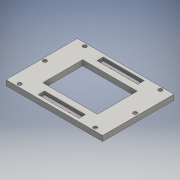
# Autodesk Inventor part: modified_xyStageMount
Saved by Autodesk Inventor 2016 (Build 200138000, 138)
## iProperties
Created: 2016-09-14
Part Number: modified_xyStageMount
Material: Generic
Document SubType Name: Modeling
Designer: sims01
Density: 1 g/cm^3
Appearance: Default
Author: sims01
Autodesk Inventor part; units mm, degrees
ref_plane "YZ Plane" through (0, 0, 0) normal (1, 0, 0) x (0, 1, 0)
ref_plane "XZ Plane" through (0, 0, 0) normal (0, 1, 0) x (-1, 0, 0)
ref_plane "XY Plane" through (0, 0, 0) normal (0, 0, 1) x (1, 0, 0)
sketch "Sketch1" plane through (0, 0, 0) normal (0, 0, 1) x (1, 0, 0)
  line L0 (-230, 170) -> (230, 170)
  line L1 (230, 170) -> (230, -170)
  line L2 (230, -170) -> (-230, -170)
  line L3 (-230, -170) -> (-230, 170)
  line L4 (130, 170) -> (230, 170)
  line L5 (230, 170) -> (230, -170)
  line L6 (230, -170) -> (130, -170)
  line L7 (130, -170) -> (130, 170)
  line L8 (-230, 170) -> (-130, 170)
  line L9 (-130, 170) -> (-130, -170)
  line L10 (-130, -170) -> (-230, -170)
  line L11 (-230, -170) -> (-230, 170)
  line L12 (-230, 170) -> (230, 170)
  line L13 (230, 170) -> (230, 95)
  line L14 (230, 95) -> (-230, 95)
  line L15 (-230, 95) -> (-230, 170)
  line L16 (-230, -95) -> (230, -95)
  line L17 (230, -95) -> (230, -170)
  line L18 (230, -170) -> (-230, -170)
  line L19 (-230, -170) -> (-230, -95)
  point P0 (0, 0)
  dimension "d0" = 460
  dimension "d1" = 340
  dimension "d2" = 170
  dimension "d3" = 230
  dimension "d4" = 100
  dimension "d5" = 100
  dimension "d6" = 75
  dimension "d7" = 75
  constraints: 40 end point, 12 collinear, 10 parallel, 5 horizontal, 5 perpendicular
  measures "d0" distance of L0.start L0.end
  measures "d1" distance of L0.end L1.end
  measures "d2" distance from line of point (0, 0) L0
  measures "d3" distance from line of point (0, 0) L1
  measures "d4" distance of L4.start L4.end
  measures "d5" distance of L8.start L8.end
  measures "d6" distance between parallel lines of L2 L16
  measures "d7" distance between parallel lines of L14 L0
extrude "Extrusion1" add sketch "Sketch1" along normal blind 25 contours L0 L9 L14 L3 | L0 L7 L14 L9 | L14 L9 L16 L3 | L0 L1 L14 L7 | L16 L9 L2 L3 | L14 L1 L16 L7 | L16 L7 L2 L9 | L16 L1 L2 L7
sketch "Sketch2" plane through (0, 0, 25) normal (0, 0, 1) x (1, 0, 0)
  line L0 (-92.0312, -155) -> (102.9688, -155)
  line L1 (102.9688, -155) -> (102.9688, -125)
  line L2 (102.9688, -125) -> (-92.0313, -125)
  line L3 (-92.0313, -125) -> (-92.0312, -155)
  line L4 (-230, -170) -> (230, -170) projected
  point P0 (0, 0)
  dimension "d10" = 30
  dimension "d11" = 195
  dimension "d12" = 15
  constraints: 8 end point, 2 parallel, 1 horizontal, 1 perpendicular
  measures "d10" distance of L2.end L0.start
  measures "d11" distance of L0.start L0.end
  measures "d12" distance between parallel lines of L4 L0
extrude "Extrusion2" cut sketch "Sketch2" against normal blind 16
sketch "Sketch3" plane through (0, 0, 9) normal (0, 0, 1) x (1, 0, 0)
  line L0 (102.9688, -155) -> (-92.0312, -155) projected
  point P0 (0, 0)
  point P1 (-40, -140)
  point P2 (40, -140)
  dimension "d15" = 15
  dimension "d16" = 80
  dimension "d17" = 40
  constraints: 1 horizontal alignment
  measures "d15" distance from line of L0 point (-40, -140)
  measures "d16" distance of point (40, -140) point (-40, -140)
  measures "d17" horizontal distance of point (-40, -140) point (0, 0)
hole "Hole1" at (-40, -140, 9) at (40, -140, 9) direction (0, 0, -1) diameter 5.5 end through all
mirror "Mirror2" about plane through (0, 0, 0) normal (0, 1, 0) of "Extrusion2", "Hole1"
sketch "Sketch4" plane through (0, 0, 25) normal (0, 0, 1) x (1, 0, 0)
  line L0 (230, -170) -> (230, 170) projected
  line L1 (230, 170) -> (-230, 170) projected
  point P0 (0, 0)
  point P1 (180, 155)
  point P2 (215, 0)
  dimension "d25" = 15
  dimension "d26" = 15
  dimension "d27" = 50
  constraints: 1 horizontal alignment
  measures "d25" distance from line of point (215, 0) L0
  measures "d26" distance from line of L1 point (180, 155)
  measures "d27" distance from line of point (180, 155) L0
hole "Hole2" at (180, 155, 25) at (215, 0, 25) direction (0, 0, -1) diameter 6.6 end through all counterbore diameter 18 counterbore depth 6.6 clearance for "Hex Head Cap Screw ISO 24017" size "M6" standard "ISO"
mirror "Mirror3" about plane through (0, 0, 0) normal (0, 1, 0) of "Hole2"
mirror "Mirror4" about plane through (0, 0, 0) normal (1, 0, 0) of "Hole2", "Mirror3"
equation "\"d2\" = 0.5 * d1"
equation "\"d3\" = 0.5 * d0"
equation "\"d17\" = 0.5 * d16"
body "Solid1"
